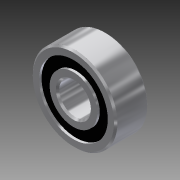
# Autodesk Inventor part: R3-2RS
Saved by Autodesk Inventor 2014 SP1 (Build 180222100, 222)
## iProperties
Created: 2013-06-25
Part Number: R3-2RS
Material: Generic
Document SubType Name: Modeling
Designer: mvarma
Density: 1 g/cm^3
Mass: 0.505242 g
Surface Area: 5.16319 cm^2
Volume: 0.505242 cm^3
Appearance: Aluminum - Polished
Author: mvarma
Autodesk Inventor part; units mm, degrees
ref_plane "YZ Plane" through (0, 0, 0) normal (1, 0, 0) x (0, 1, 0)
ref_plane "XZ Plane" through (0, 0, 0) normal (0, 1, 0) x (-1, 0, 0)
ref_plane "XY Plane" through (0, 0, 0) normal (0, 0, 1) x (1, 0, 0)
sketch "Sketch1" plane through (0, 0, 0) normal (0, 0, 1) x (1, 0, 0)
  circle A0 centre (0, 0) radius 6.35
  circle A1 centre (0, 0) radius 2.3813
  circle A2 centre (0, 0) radius 3.5719
  circle A3 centre (0, 0) radius 5.1594
  dimension "d0" = 12.7
  dimension "d1" = 4.7625
  dimension "d2" = 7.1437
  dimension "d3" = 10.3187
  constraints: 4 centre point, 4 coincident
  measures "d0" diameter of A0
  measures "d1" diameter of A1
  measures "d2" diameter of A2
  measures "d3" diameter of A3
extrude "Extrusion1" add sketch "Sketch1" along normal blind 2.4892
extrude "Extrusion2" add sketch "Sketch1" along normal blind 2.1082 contours A3
chamfer "Chamfer1" distance 0.254 angle 45 2 edges at (-6.35, 0, 2.4892) (-2.3813, 0, 2.4892)
mirror "Mirror1" about plane through (0, 0, 0) normal (0, 0, -1)
body "Solid1"
